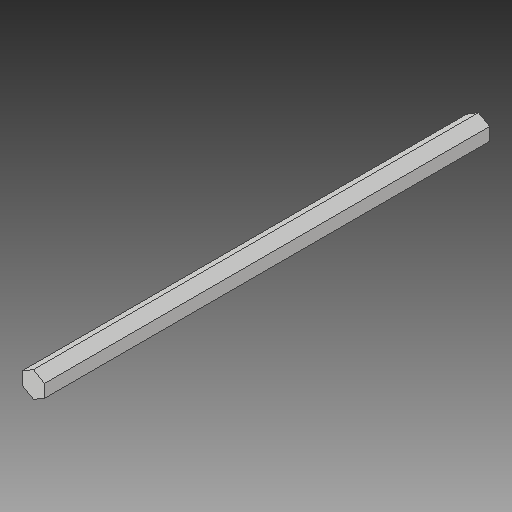
# Autodesk Inventor part: Hex Shaft
Saved by Autodesk Inventor 2018 (Build 220112000, 112)
## iProperties
Created: 2019-01-18
Part Number: Hex Shaft
Material: Generic
Document SubType Name: Modeling
Designer: Gabriel
Density: 1 g/cm^3
Appearance: Default
Author: Gabriel
Autodesk Inventor part; units mm, degrees
ref_plane "YZ Plane" through (0, 0, 0) normal (1, 0, 0) x (0, 1, 0)
ref_plane "XZ Plane" through (0, 0, 0) normal (0, 1, 0) x (-1, 0, 0)
ref_plane "XY Plane" through (0, 0, 0) normal (0, 0, 1) x (1, 0, 0)
sketch "Sketch1" plane through (0, 0, 0) normal (0, 0, 1) x (1, 0, 0)
  line L0 (-1.9536, 0.6855) -> (4.3964, 0.6855)
  line L1 (4.3964, -2.9551) -> (-1.9315, -6.6341)
  line L2 (-1.9315, -6.6341) -> (-8.2815, -2.9935)
  line L3 (-8.2815, -2.9935) -> (-8.3036, 4.3261)
  line L4 (-8.3036, 4.3261) -> (-1.9757, 8.0051)
  line L5 (-1.9757, 8.0051) -> (4.3743, 4.3644)
  line L6 (4.3743, 4.3644) -> (4.3964, -2.9551)
  dimension "d0" = 6.35
  constraints: 14 end point, 1 coincident, 1 horizontal, 13 other
  measures "d0" distance of L0.start L0.end
extrude "Extrusion1" add sketch "Sketch1" along normal blind 254
body "Solid1"
